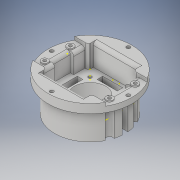
# Autodesk Inventor part: Corona_Cam_Mount_v7
Saved by Autodesk Inventor 2018 (Build 220112000, 112)
## iProperties
Created: 2020-03-31
Part Number: Corona_Cam_Mount_v7
Material: Generic
Document SubType Name: Modeling
Designer: Ian
Density: 1 g/cm^3
Appearance: Default
Author: Ian
Autodesk Inventor part; units mm, degrees
ref_plane "YZ Plane" through (0, 0, 0) normal (1, 0, 0) x (0, 1, 0)
ref_plane "XZ Plane" through (0, 0, 0) normal (0, 1, 0) x (-1, 0, 0)
ref_plane "XY Plane" through (0, 0, 0) normal (0, 0, 1) x (1, 0, 0)
sketch "Sketch1" plane through (0, 0, 0) normal (0, 1, 0) x (-1, 0, 0)
  circle A0 centre (0, -34.29) radius 1.651
  circle A1 centre (-34.29, 0) radius 1.651
  circle A2 centre (0, 34.29) radius 1.651
  circle A3 centre (34.29, 0) radius 1.651
  circle A4 centre (0, 0) radius 37.465
  circle A5 centre (0, 0) radius 31.6865
  circle A6 centre (13.97, -13.97) radius 1.27
  circle A7 centre (-13.97, -13.97) radius 1.27
  circle A8 centre (13.97, 13.97) radius 1.27
  circle A9 centre (-13.97, 13.97) radius 1.27
  line L0 (18.161, -18.161) -> (-18.161, -18.161)
  line L1 (-18.161, -18.161) -> (-18.161, 18.161)
  line L2 (-18.161, 18.161) -> (18.161, 18.161)
  line L3 (18.161, 18.161) -> (18.161, -18.161)
  circle A10 centre (0, 0) radius 13.97
  line L4 (18.161, -20.161) -> (20.161, -20.161)
  line L5 (20.161, -20.161) -> (-18.161, -20.161)
  line L6 (-18.161, -20.161) -> (-20.161, -20.161)
  line L7 (-20.161, -20.161) -> (-20.161, 18.161)
  line L8 (-20.161, 18.161) -> (-20.161, 20.161)
  line L9 (-20.161, 20.161) -> (18.161, 20.161)
  line L10 (20.161, -20.161) -> (20.161, 20.161)
  line L11 (20.161, 20.161) -> (18.161, 20.161)
  dimension "d3" = 2
  dimension "d4" = 2
  dimension "d5" = 2
  constraints: 24 end point, 11 centre point, 5 perpendicular, 3 point on line, 1 coincident, 1 horizontal, 1 vertical
  measures "d3" distance of L4.start L4.end
  measures "d4" distance of L5.end L6.end
  measures "d5" distance of L7.end L8.end
extrude "Extrusion1" add sketch "Sketch1" against normal blind 10 contours A4 | A5 | L0 L1 L2 L3 | L5 L6 L7 L8 L9 L11 L10 L4
extrude "Extrusion2" cut sketch "Sketch1" against normal blind 5 contours L0 L1 L2 L3 | L5 L6 L7 L8 L9 L11 L10 L4
sketch "Sketch2" plane through (0, -10, 0) normal (0, -1, 0) x (1, 0, 0)
  circle A0 centre (0, 0) radius 13.9624
  circle A1 centre (0, 0) radius 23
  circle A2 centre (0, 0) radius 31.5
  circle A3 centre (0, 0) radius 15
  dimension "d11" = 46
  dimension "d13" = 63
  dimension "d14" = 30
  constraints: 4 centre point, 3 coincident
  measures "d11" diameter of A1
  measures "d13" diameter of A2
  measures "d14" diameter of A3
extrude "Extrusion3" add sketch "Sketch2" along normal blind 26 contours A1
extrude "Extrusion4" add sketch "Sketch2" along normal blind 26
sketch "Sketch3" plane through (0, -5, 0) normal (0, 1, 0) x (1, 0, 0)
  circle A0 centre (-13.97, 13.97) radius 1.27 projected
  circle A1 centre (-13.97, 13.97) radius 1.4
  circle A2 centre (13.97, 13.97) radius 1.27 projected
  circle A3 centre (13.97, 13.97) radius 1.4
  circle A4 centre (13.97, -13.97) radius 1.27 projected
  circle A5 centre (13.97, -13.97) radius 1.4
  circle A6 centre (-13.97, -13.97) radius 1.27 projected
  circle A7 centre (-13.97, -13.97) radius 1.4
  point P0 (0, 0)
  dimension "d19" = 2.8
  dimension "d20" = 2.8
  dimension "d21" = 2.8
  dimension "d22" = 2.8
  constraints: 4 centre point, 4 coincident
  measures "d19" diameter of A1
  measures "d20" diameter of A3
  measures "d21" diameter of A5
  measures "d22" diameter of A7
extrude "Extrusion5" cut sketch "Sketch3" against normal blind 50 contours A0 | A1 | A2 | A3 | A4 | A5 | A6 | A7
sketch "Sketch4" plane through (0, -36, 0) normal (0, -1, 0) x (1, 0, 0)
  circle A0 centre (13.97, 13.97) radius 1.4 projected
  circle A1 centre (13.97, 13.97) radius 2.75
  circle A2 centre (13.97, -13.97) radius 1.4 projected
  circle A3 centre (13.97, -13.97) radius 2.75
  circle A4 centre (-13.97, 13.97) radius 1.4 projected
  circle A5 centre (-13.97, 13.97) radius 2.75
  circle A6 centre (-13.97, -13.97) radius 1.4 projected
  circle A7 centre (-13.97, -13.97) radius 2.75
  point P0 (0, 0)
  dimension "d25" = 5.5
  dimension "d26" = 5.5
  dimension "d27" = 5.5
  dimension "d28" = 5.5
  constraints: 4 centre point, 4 coincident
  measures "d25" diameter of A1
  measures "d26" diameter of A3
  measures "d27" diameter of A5
  measures "d28" diameter of A7
extrude "Extrusion6" cut sketch "Sketch4" against normal blind 11
sketch "Sketch5" plane through (0, -36, 0) normal (0, -1, 0) x (1, 0, 0)
  circle A0 centre (13.97, 13.97) radius 1.4 projected
  circle A1 centre (13.97, -13.97) radius 1.4 projected
  line L0 (15.37, 8.97) -> (20.37, 8.97)
  line L1 (15.37, -8.97) -> (20.37, -8.97)
  line L2 (20.37, -8.97) -> (20.37, 8.97)
  line L3 (15.37, 8.97) -> (15.37, -8.97)
  circle A2 centre (0, 0) radius 13.97 projected
  circle A3 centre (-13.97, -13.97) radius 1.4 projected
  line L4 (8.97, -15.37) -> (8.97, -20.37)
  line L5 (-8.97, -15.37) -> (-8.97, -20.37)
  line L6 (-8.97, -20.37) -> (8.97, -20.37)
  line L7 (8.97, -15.37) -> (-8.97, -15.37)
  line L8 (-15.37, 8.97) -> (-20.37, 8.97)
  line L9 (-15.37, -8.97) -> (-20.37, -8.97)
  line L10 (-20.37, -8.97) -> (-20.37, 8.97)
  line L11 (-15.37, 8.97) -> (-15.37, -8.97)
  line L12 (8.97, 15.37) -> (8.97, 20.37)
  line L13 (-8.97, 15.37) -> (-8.97, 20.37)
  line L14 (-8.97, 20.37) -> (8.97, 20.37)
  line L15 (8.97, 15.37) -> (-8.97, 15.37)
  dimension "d32" = 5
  dimension "d34" = 5
  constraints: 32 end point, 1 horizontal, 1 perpendicular, 1 vertical
  measures "d32" distance of L0.start L0.end
  measures "d34" distance of L1.start L1.end
extrude "Extrusion7" cut sketch "Sketch5" against normal blind 50 contours L0 L2 L1 L3 | L4 L6 L5 L7 | L11 L9 L10 L8 | L15 L13 L14 L12
sketch "Sketch6" plane through (0, -5, 0) normal (0, 1, 0) x (1, 0, 0)
  line L0 (8.97, 20.161) -> (20.161, 20.161) projected
  line L1 (20.161, -20.161) -> (8.97, -20.161) projected
  line L2 (20.161, 20.161) -> (20.161, -20.161)
  line L3 (-20.161, -20.161) -> (-20.161, -8.97) projected
  line L4 (20.161, -20.161) -> (-20.161, -20.161)
  line L5 (-20.161, 8.97) -> (-20.161, 20.161) projected
  line L6 (-20.161, -20.161) -> (-20.161, 20.161)
  line L7 (-20.161, 20.161) -> (20.161, 20.161)
  point P0 (0, 0)
  constraints: 8 end point, 3 perpendicular, 1 vertical
extrude "Extrusion8" cut sketch "Sketch6" against normal blind 17
sketch "Sketch21" plane through (0, 0, 0) normal (0, 1, 0) x (1, 0, 0)
  line L0 (-29, 0) -> (-29, 11.5)
  line L1 (-29, 11.5) -> (29, 11.5)
  line L2 (29, 11.5) -> (29, -11.5)
  line L3 (29, -11.5) -> (-29, -11.5)
  line L4 (-29, -11.5) -> (-29, 0)
  circle A0 centre (0, 0) radius 37.465 projected
  line L5 (32.5, -15) -> (34.3311, -15)
  line L6 (32.5, -15) -> (32.5, -18.638)
  line L7 (-32.5, 18.638) -> (32.5, 18.638)
  line L8 (32.5, -18.638) -> (-32.5, -18.638)
  arc A1 (-32.5, 18.638) -> (-32.5, -18.638) centre (0, 0) ccw
  arc A2 (32.5, -18.638) -> (32.5, 18.638) centre (0, 0) ccw
  circle A3 centre (-29, 11.5) radius 1.4
  circle A4 centre (29, 11.5) radius 1.4
  circle A5 centre (29, -11.5) radius 1.4
  circle A6 centre (-29, -11.5) radius 1.4
  dimension "d132" = 2.8
  dimension "d133" = 2.8
  dimension "d134" = 2.8
  dimension "d135" = 2.8
  constraints: 18 end point, 9 point on circle, 6 centre point, 5 coincident, 2 perpendicular, 1 horizontal, 1 parallel, 1 point on line
  measures "d132" diameter of A3
  measures "d133" diameter of A4
  measures "d134" diameter of A5
  measures "d135" diameter of A6
sketch "Sketch22" plane through (0, 0, 0) normal (0, 1, 0) x (1, 0, 0)
  circle A0 centre (0, 0) radius 37.465
  constraints: 1 centre point, 1 coincident
extrude "Extrusion21" cut sketch "Sketch22" against normal blind 2
extrude "Extrusion22" cut sketch "Sketch21" against normal blind 5 contours L0 A3 L1 A4 L2 A5 L3 A6 L4 | A3 L1 L0 | L0 L1 A3 | A6 L3 L4 | L4 L3 A6 | A4 L2 L1 | L1 L2 A4 | A5 L2 L3 | L3 L2 A5 | A0 L5 L6 L8 L7 | A0 L6 L5
sketch "Sketch23" plane through (0, -5, 0) normal (0, 1, 0) x (1, 0, 0)
  circle A0 centre (-29, 11.5) radius 1.4
  circle A1 centre (29, 11.5) radius 1.4
  circle A2 centre (29, -11.5) radius 1.4
  circle A3 centre (-29, -11.5) radius 1.4
  dimension "d138" = 2.8
  dimension "d139" = 2.8
  dimension "d140" = 2.8
  dimension "d141" = 2.8
  constraints: 4 centre point
  measures "d138" diameter of A0
  measures "d139" diameter of A1
  measures "d140" diameter of A2
  measures "d141" diameter of A3
extrude "Extrusion23" cut sketch "Sketch23" against normal blind 50
sketch "Sketch24" plane through (0, -36, 0) normal (0, -1, 0) x (1, 0, 0)
  arc A0 (-28.7477, -12.8771) -> (-29.76, -10.3243) centre (-29, -11.5) ccw projected
  circle A1 centre (-29, -11.5) radius 4.5
  arc A2 (29.76, -10.3243) -> (28.7477, -12.8771) centre (29, -11.5) ccw projected
  circle A3 centre (29, -11.5) radius 4.5
  circle A4 centre (-29, 11.5) radius 1.4 projected
  circle A5 centre (-29, 11.5) radius 4.5
  circle A6 centre (29, 11.5) radius 1.4 projected
  circle A7 centre (29, 11.5) radius 4.5
  point P0 (0, 0)
  dimension "d145" = 9
  dimension "d146" = 9
  dimension "d147" = 9
  dimension "d148" = 9
  constraints: 4 centre point, 4 coincident
  measures "d145" diameter of A1
  measures "d146" diameter of A3
  measures "d147" diameter of A5
  measures "d148" diameter of A7
extrude "Extrusion24" cut sketch "Sketch24" against normal blind 29
sketch "Sketch25" plane through (0, -36, 0) normal (0, -1, 0) x (1, 0, 0)
  circle A0 centre (13.97, 13.97) radius 1.4 projected
  circle A1 centre (13.97, 13.97) radius 3
  circle A2 centre (13.97, -13.97) radius 1.4 projected
  circle A3 centre (13.97, -13.97) radius 3
  circle A4 centre (-13.97, -13.97) radius 1.4 projected
  circle A5 centre (-13.97, -13.97) radius 3
  circle A6 centre (-13.97, 13.97) radius 1.4 projected
  circle A7 centre (-13.97, 13.97) radius 3
  point P0 (0, 0)
  dimension "d151" = 6
  dimension "d152" = 6
  dimension "d153" = 6
  dimension "d154" = 6
  constraints: 4 centre point, 4 coincident
  measures "d151" diameter of A1
  measures "d152" diameter of A3
  measures "d153" diameter of A5
  measures "d154" diameter of A7
extrude "Extrusion25" cut sketch "Sketch25" against normal blind 11
sketch "Sketch26" plane through (0, -5, 0) normal (0, 1, 0) x (1, 0, 0)
  line L0 (20.161, 18.638) -> (32.5, 18.638) projected
  line L1 (20.161, 18.638) -> (23.161, 18.638)
  line L2 (23.161, 18.638) -> (23.161, -18.638)
  line L3 (32.5, -18.638) -> (20.161, -18.638) projected
  line L4 (20.161, -18.638) -> (20.161, 18.638)
  line L5 (20.161, -18.638) -> (20.161, -8.97) projected
  line L6 (23.161, -18.638) -> (20.161, -18.638)
  point P0 (0, 0)
  dimension "d157" = 3
  constraints: 8 end point, 2 point on line, 1 horizontal, 1 parallel, 1 perpendicular
  measures "d157" distance of L0.start L1.end
extrude "Extrusion26" cut sketch "Sketch26" against normal blind 17
sketch "Sketch27" plane through (0, -5, 0) normal (0, 1, 0) x (1, 0, 0)
  line L0 (-32.5, 18.638) -> (-20.161, 18.638) projected
  line L1 (-20.161, 18.638) -> (-23.161, 18.638)
  line L2 (-23.161, 18.638) -> (-23.161, -18.638)
  line L3 (-20.161, -18.638) -> (-32.5, -18.638) projected
  line L4 (-20.161, -18.638) -> (-23.161, -18.638)
  line L5 (-20.161, -18.638) -> (-20.161, 18.638)
  line L6 (-20.161, 8.97) -> (-20.161, 20.161) projected
  point P0 (0, 0)
  dimension "d160" = 3
  constraints: 8 end point, 2 perpendicular, 2 point on line, 1 collinear
  measures "d160" distance of L0.end L1.end
extrude "Extrusion27" cut sketch "Sketch27" against normal blind 17
sketch "Sketch28" plane through (0, -2, 0) normal (0, 1, 0) x (1, 0, 0)
  line L0 (20.161, 20.161) -> (20.161, 18.638) projected
  line L1 (20.161, 20.161) -> (20.161, 23.161)
  line L2 (-20.1219, 20.161) -> (20.161, 20.161)
  line L3 (20.161, 23.161) -> (-20.1219, 23.161)
  line L4 (-20.1219, 23.161) -> (-20.1219, 20.161)
  point P0 (0, 0)
  dimension "d163" = 3
  constraints: 8 end point, 2 horizontal, 1 perpendicular, 1 vertical
  measures "d163" distance of L0.start L1.end
extrude "Extrusion28" cut sketch "Sketch28" against normal blind 20
sketch "Sketch29" plane through (0, -2, 0) normal (0, 1, 0) x (1, 0, 0)
  line L0 (20.161, -20.161) -> (20.161, -23.161)
  line L1 (-8.97, -20.161) -> (-20.161, -20.161) projected
  line L2 (20.161, -20.161) -> (-20.161, -20.161)
  line L3 (-20.161, -20.161) -> (-20.161, -23.161)
  line L4 (-20.161, -23.161) -> (20.161, -23.161)
  point P0 (0, 0)
  dimension "d166" = 3
  constraints: 8 end point, 2 perpendicular, 1 horizontal, 1 vertical
  measures "d166" distance of L0.start L0.end
extrude "Extrusion29" cut sketch "Sketch29" against normal blind 20
fillet "Fillet4" radius 3 2 edges at (20.161, -12, -18.638) (20.161, -12, 18.638)
fillet "Fillet5" radius 3 1 edges at (23.161, -5, 0)
fillet "Fillet6" radius 3 3 edges at (-20.161, -12, -18.638) (-20.161, -12, 18.638) (-23.161, -5, 0)
sketch "Sketch30" plane through (0, -36, 0) normal (0, -1, 0) x (1, 0, 0)
  circle A0 centre (0, 0) radius 13.9624
  circle A1 centre (0, 0) radius 15
  circle A2 centre (0, 0) radius 23
  dimension "d172" = 30
  dimension "d173" = 46
  constraints: 3 centre point, 3 coincident
  measures "d172" diameter of A1
  measures "d173" diameter of A2
extrude "Extrusion30" cut sketch "Sketch30" against normal blind 4.5 contours A2
sketch "Sketch32" plane through (0, -2, 0) normal (0, 1, 0) x (1, 0, 0)
  point P0 (0, 0)
sketch "Sketch33" plane through (0, -5, 0) normal (0, 1, 0) x (1, 0, 0)
  circle A0 centre (-29, -11.5) radius 1.4 projected
  line L0 (-23.161, -18.638) -> (-32.5, -18.638) projected
  line L1 (-26.6, -18.638) -> (-23.161, -18.638)
  line L2 (-23.161, -18.638) -> (-23.161, 18.638)
  line L3 (-26.161, 18.638) -> (-26.161, -18.638) projected
  line L4 (-23.161, 18.638) -> (-22.7722, 18.638) projected
  line L5 (-26.6, 18.638) -> (-23.161, 18.638)
  line L6 (-23.161, 0) -> (-23.161, -9)
  line L7 (-23.161, -18.638) -> (-23.161, 18.638) projected
  circle A1 centre (-29, -11.5) radius 3
  line L8 (-23.161, -9) -> (-23.161, -8.5)
  line L9 (-23.161, 10) -> (-23.161, 9.5)
  line L10 (-26.161, -8.5) -> (-26.161, 8.5)
  line L11 (-23.161, 0) -> (-23.161, -8.5)
  line L12 (-23.161, 0) -> (-23.161, 8.5)
  line L13 (-23.161, 8.5) -> (-26.161, 8.5)
  line L14 (-26.161, -8.5) -> (-23.161, -8.5)
  point P0 (0, 0)
  dimension "d198" = 6
  dimension "d200" = 0.5
  dimension "d215" = 8.5
  dimension "d216" = 8.5
  constraints: 22 end point, 7 point on line, 2 perpendicular, 1 centre point, 1 coincident, 1 collinear, 1 horizontal, 1 midpoint
  measures "d198" diameter of A1
  measures "d200" distance of L9.start L9.end
  measures "d215" distance of L6.start L8.end
  measures "d216" distance of L6.start L12.end
sketch "Sketch34" plane through (-29, -7, -11.5) normal (0, -1, 0) x (1, 0, 0)
  point P0 (29, 11.5)
sketch "Sketch35" plane through (-29, -7, -11.5) normal (0, -1, 0) x (1, 0, 0)
  arc A0 (0.9553, -2.8438) -> (-1.2533, 2.7257) centre (0, 0) ccw
  arc A1 (1.6774, -4.1757) -> (-1.6402, 4.1904) centre (0, 0) ccw
  arc A2 (-1.6402, 4.1904) -> (1.6774, -4.1757) centre (29, 11.5) ccw
  dimension "d185" = 6
  dimension "d186" = 9
  constraints: 8 point on circle, 3 centre point, 2 coincident
  measures "d185" diameter of A0
  measures "d186" diameter of A1
extrude "Extrusion32" add sketch "Sketch35" along normal blind 29 contours A0 A2 A1
sketch "Sketch36" plane through (-29, -7, 11.5) normal (0, -1, 0) x (1, 0, 0)
  arc A0 (1.6774, 4.1757) -> (-1.6402, -4.1904) centre (29, -11.5) ccw
  arc A1 (-1.2533, -2.7257) -> (0.9553, 2.8438) centre (0, 0) ccw
  arc A2 (-1.6402, -4.1904) -> (1.6774, 4.1757) centre (0, 0) ccw
  dimension "d189" = 6
  constraints: 8 point on circle, 3 centre point, 2 coincident
  measures "d189" diameter of A1
extrude "Extrusion33" add sketch "Sketch36" along normal blind 29 contours A2 A0 A1
sketch "Sketch37" plane through (29, -7, 11.5) normal (0, -1, 0) x (1, 0, 0)
  arc A0 (-0.9553, 2.8438) -> (1.2533, -2.7257) centre (0, 0) ccw
  arc A1 (-1.6774, 4.1757) -> (1.6402, -4.1904) centre (0, 0) ccw
  arc A2 (1.6402, -4.1904) -> (-1.6774, 4.1757) centre (-29, -11.5) ccw
  dimension "d192" = 6
  constraints: 8 point on circle, 3 centre point, 2 coincident
  measures "d192" diameter of A0
extrude "Extrusion34" add sketch "Sketch37" along normal blind 29 contours A0 A2 A1
sketch "Sketch38" plane through (29, -7, -11.5) normal (0, -1, 0) x (1, 0, 0)
  arc A0 (1.2533, 2.7257) -> (-0.9553, -2.8438) centre (0, 0) ccw
  arc A1 (1.6402, 4.1904) -> (-1.6774, -4.1757) centre (0, 0) ccw
  arc A2 (-1.6774, -4.1757) -> (1.6402, 4.1904) centre (-29, 11.5) ccw
  dimension "d195" = 6
  constraints: 8 point on circle, 3 centre point, 2 coincident
  measures "d195" diameter of A0
extrude "Extrusion35" add sketch "Sketch38" along normal blind 29 contours A0 A2 A1
sketch "Sketch39" plane through (0, -5, 0) normal (0, 1, 0) x (1, 0, 0)
  line L0 (23.161, 18.638) -> (23.161, -18.638) projected
  line L1 (23.161, 0) -> (23.161, -8.5)
  arc A0 (30.2533, -8.7743) -> (30.2533, 8.7743) centre (0, 0) ccw projected
  line L2 (23.161, 0) -> (23.161, 8.5)
  line L3 (23.161, -8.5) -> (26.161, -8.5)
  line L4 (26.161, -18.638) -> (26.161, 18.638) projected
  line L5 (26.161, -8.5) -> (26.161, 8.5)
  line L6 (26.161, 8.5) -> (23.161, 8.5)
  line L7 (27.161, 8.5) -> (26.161, 8.5)
  dimension "d204" = 8.5
  dimension "d208" = 3
  constraints: 12 end point, 4 point on line, 1 collinear, 1 midpoint, 1 perpendicular
  measures "d204" distance of L1.start L1.end
  measures "d208" distance of L1.end L3.end
extrude "Extrusion37" cut sketch "Sketch39" against normal blind 17
fillet "Fillet8" radius 3 1 edges at (26.161, -5, 0)
extrude "Extrusion38" cut sketch "Sketch33" against normal blind 17 contours L14 L3 L13 L2
fillet "Fillet9" radius 3 1 edges at (-26.161, -5, 0)
sketch "Sketch40" plane through (0, -5, 0) normal (0, 1, 0) x (1, 0, 0)
  circle A0 centre (-29, 11.5) radius 1.4 projected
  circle A1 centre (-29, 11.5) radius 1.4
  circle A2 centre (-29, 11.5) radius 3
  circle A3 centre (-29, -11.5) radius 1.4 projected
  circle A4 centre (-29, -11.5) radius 1.4
  circle A5 centre (-29, -11.5) radius 3
  point P0 (0, 0)
  dimension "d220" = 6
  dimension "d221" = 6
  constraints: 4 centre point, 4 coincident
  measures "d220" diameter of A2
  measures "d221" diameter of A5
extrude "Extrusion39" add sketch "Sketch40" along normal blind 1
sketch "Sketch41" plane through (0, -5, 0) normal (0, 1, 0) x (1, 0, 0)
  circle A0 centre (29, 11.5) radius 1.4 projected
  circle A1 centre (29, 11.5) radius 1.4
  circle A2 centre (29, 11.5) radius 3
  circle A3 centre (29, -11.5) radius 1.4 projected
  circle A4 centre (29, -11.5) radius 1.4
  circle A5 centre (29, -11.5) radius 3
  point P0 (0, 0)
  dimension "d224" = 6
  dimension "d225" = 6
  constraints: 4 centre point, 4 coincident
  measures "d224" diameter of A2
  measures "d225" diameter of A5
extrude "Extrusion40" add sketch "Sketch41" along normal blind 1
sketch "Sketch42" plane through (0, -22, 0) normal (0, 1, 0) x (1, 0, 0)
  circle A0 centre (13.97, 13.97) radius 1.4 projected
  circle A1 centre (13.97, 13.97) radius 1.5
  circle A2 centre (13.97, -13.97) radius 1.4 projected
  circle A3 centre (13.97, -13.97) radius 1.5
  circle A4 centre (-13.97, -13.97) radius 1.4 projected
  circle A5 centre (-13.97, -13.97) radius 1.5
  circle A6 centre (-13.97, 13.97) radius 1.4 projected
  circle A7 centre (-13.97, 13.97) radius 1.5
  point P0 (0, 0)
  dimension "d228" = 3
  dimension "d229" = 3
  dimension "d230" = 3
  dimension "d231" = 3
  constraints: 4 centre point, 4 coincident
  measures "d228" diameter of A1
  measures "d229" diameter of A3
  measures "d230" diameter of A5
  measures "d231" diameter of A7
extrude "Extrusion41" cut sketch "Sketch42" against normal blind 5
fillet "Fillet10" radius 3 2 edges at (0.0195, -2, -23.161) (0, -2, 23.161)
sketch "Sketch43" plane through (0, -10, 0) normal (0, -1, 0) x (1, 0, 0)
  point P0 (0, 0)
sketch "Sketch44" plane through (20.37, -22, -8.97) normal (-1, 0, 0) x (0, 0, 1)
  point P0 (8.97, 22)
sketch "Sketch45" plane through (26.161, -22, -8.5) normal (-1, 0, 0) x (0, 0, 1)
  line L0 (22.4624, 0) -> (-5.4624, 0) projected
  line L1 (8.5, 0) -> (18.5, 0) construction
  point P0 (8.5, 22)
  constraints: 2 end point, 1 horizontal, 1 midpoint
sketch "Sketch46" plane through (-20.37, -22, 8.97) normal (1, 0, 0) x (0, 0, -1)
  point P0 (8.97, 22)
sketch "Sketch47" plane through (0, -22, 0) normal (0, 1, 0) x (1, 0, 0)
  line L0 (15.37, -2.5) -> (13.7368, -2.5)
  circle A0 centre (0, 0) radius 13.9624 projected
  line L1 (13.7368, 2.5) -> (13.7368, -2.5)
  line L2 (13.7368, 2.5) -> (15.37, 2.5)
  line L3 (15.37, 2.5) -> (37.3815, 2.5)
  arc A1 (32.5, -18.638) -> (32.5, 18.638) centre (0, 0) ccw projected
  line L4 (15.37, -2.5) -> (37.3815, -2.5)
  arc A2 (37.3815, -2.5) -> (37.3815, 2.5) centre (0, 0) ccw
  constraints: 10 end point, 5 point on circle, 2 point on line, 1 centre point, 1 coincident, 1 perpendicular
extrude "Extrusion42" cut sketch "Sketch47" against normal blind 14 and the other way blind 10 contours L0 A0 L2 L3 A1 L4
body "Solid1"
